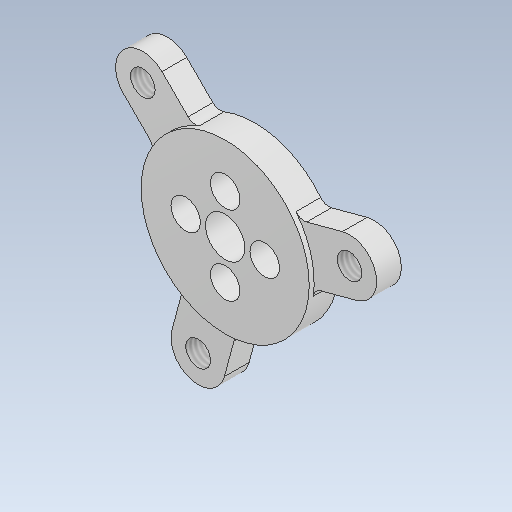
# Autodesk Inventor part: 脚中間フレームカム3
Saved by Autodesk Inventor 2020.2 (Build 242310000, 310)
## iProperties
Created: 2020-03-13
Part Number: 脚中間フレームカム3
Material: アルミニウム 2014-T4
Document SubType Name: Modeling
Designer: aoyam
Density: 2.8 g/cm^3
Appearance: サテン
Mass: 2.19522 g
Surface Area: 10.0909 cm^2
Volume: 0.784008 cm^3
Author: aoyam
Autodesk Inventor part; units mm, degrees
ref_plane "YZ Plane" through (0, 0, 0) normal (1, 0, 0) x (0, 1, 0)
ref_plane "XZ Plane" through (0, 0, 0) normal (0, 1, 0) x (-1, 0, 0)
ref_plane "XY Plane" through (0, 0, 0) normal (0, 0, 1) x (1, 0, 0)
sketch "スケッチ1" plane through (0, 0, 0) normal (0, 0, 1) x (1, 0, 0)
  line L0 (0, 0) -> (-4, 0) construction
  circle A0 centre (-4, 0) radius 1.495
  line L1 (0, 0) -> (0, -4) construction
  circle A1 centre (0, -4) radius 1.495
  line L2 (0, 0) -> (4, 0) construction
  circle A2 centre (4, 0) radius 1.495
  line L3 (0, 0) -> (0, 4) construction
  circle A3 centre (0, 4) radius 1.495
  line L4 (0, 0) -> (-8.8388, 8.8388) construction
  circle A4 centre (-8.8388, 8.8388) radius 1.25
  line L5 (0, 0) -> (-3.2352, -12.0741) construction
  circle A5 centre (-3.2352, -12.0741) radius 1.25
  line L6 (0, 0) -> (12.0741, 3.2352) construction
  circle A6 centre (12.0741, 3.2352) radius 1.25
  circle A7 centre (0, 0) radius 8.5
  circle A8 centre (0, 0) radius 15.25
  circle A9 centre (0, 0) radius 1.995
  line L7 (0, 0) -> (-8.8388, 8.8388) construction
  line L8 (1.9445, 1.9445) -> (-6.8943, 10.7834)
  line L9 (-10.7834, 6.8943) -> (-1.9445, -1.9445)
  arc A10 (-1.9445, -1.9445) -> (1.9445, 1.9445) centre (0, 0) ccw
  arc A11 (-6.8943, 10.7834) -> (-10.7834, 6.8943) centre (-8.8388, 8.8388) ccw
  arc A12 (-5.8915, -11.3623) -> (-0.5789, -12.7858) centre (-3.2352, -12.0741) ccw
  line L10 (-2.6563, 0.7118) -> (-5.8915, -11.3623)
  line L11 (-0.5789, -12.7858) -> (2.6563, -0.7118)
  arc A13 (12.7858, 0.5789) -> (11.3623, 5.8915) centre (12.0741, 3.2352) ccw
  line L12 (0.7118, -2.6563) -> (12.7858, 0.5789)
  line L13 (11.3623, 5.8915) -> (-0.7118, 2.6563)
  point P0 (-4.4194, 4.4194)
  point P1 (-7.6317, 3.7426)
  point P2 (-4.7379, -7.057)
  point P3 (0.5747, -8.4806)
  point P4 (8.4806, -0.5747)
  point P5 (7.057, 4.7379)
  point P6 (-3.7426, 7.6317)
  dimension "d0" = 4
  dimension "d1" = 2.99
  dimension "d4" = 360
  dimension "d6" = 12.5
  dimension "d7" = 2.5
  dimension "d8" = 45
  dimension "d11" = 360
  dimension "d13" = 3.005
  dimension "d14" = 17
  dimension "d15" = 1.5
  dimension "d16" = 3.99
  dimension "d31" = 5.5
  dimension "d34" = 360
  constraints: 30 end point, 14 centre point, 11 coincident, 8 point on circle, 4 tangent, 1 horizontal, 1 midpoint, 1 parallel, 60 other
  measures "d0" distance of L0.start L0.end
  measures "d1" diameter of A0
  measures "d6" distance of L3.start L4.end
  measures "d7" diameter of A4
  measures "d8" angle of L4 L0
  measures "d14" diameter of A7
  measures "d16" diameter of A9
  measures "d31" diameter of A11
extrude "押し出し1" add sketch "スケッチ1" along normal blind 0.5 contours A0 L9 A7 L8 A3 A10 A2 A1 | L9 A10 A1 L12 L11 A7 L10 A0 | A0 L10 A7 L9 | A7 L13 A3 L8 | L11 L12 A7 | A7 L12 L11 A10 A2 L8 A3 L13 | L12 A10 L11
extrude "押し出し3" add sketch "スケッチ1" against normal blind 2.5 contours A0 L9 A7 L8 A3 A10 A2 A1 | L9 A10 A1 L12 L11 A7 L10 A0 | A0 L10 A7 L9 | L9 A11 L8 A7 | A7 L11 A12 L10 | A7 L13 A3 L8 | L11 L12 A7 | L13 A13 L12 A7 | A7 L12 L11 A10 A2 L8 A3 L13 | L12 A10 L11
thread "ねじ1" size "M3x0.5" class "6H" standard "ANSI Metric M Profile" full length
thread "ねじ2" size "M3x0.5" class "6H" standard "ANSI Metric M Profile" full length
thread "ねじ3" size "M3x0.5" class "6H" standard "ANSI Metric M Profile" full length
fillet "フィレット1" radius 1.05 6 edges at (-7.6317, 3.7426, -1.25) (-4.7379, -7.057, -1.25) (-3.7426, 7.6317, -1.25) (7.057, 4.7379, -1.25) (8.4806, -0.5747, -1.25) (0.5747, -8.4806, -1.25)
